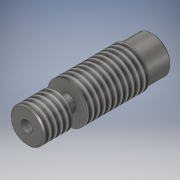
# Autodesk Inventor part: E3D-v6 1.75mm Heat Break
Saved by Autodesk Inventor 2018.2 (Build 222227000, 227)
## iProperties
Created: 2018-02-27
Part Number: E3D-v6 1.75mm Heat Break
Material: Edelstahl, 440C
Document SubType Name: Modeling
Designer: Till
Density: 7.75 g/cm^3
Appearance: Halbpoliert
Author: Till
Autodesk Inventor part; units mm, degrees
ref_plane "YZ Plane" through (0, 0, 0) normal (1, 0, 0) x (0, 1, 0)
ref_plane "XZ Plane" through (0, 0, 0) normal (0, 1, 0) x (-1, 0, 0)
ref_plane "XY Plane" through (0, 0, 0) normal (0, 0, 1) x (1, 0, 0)
sketch "Skizze1" plane through (0, 0, 0) normal (0, 0, 1) x (1, 0, 0)
  line L0 (1, 0) -> (1, 17.2649)
  line L1 (1, 17.2649) -> (2.1, 17.9)
  line L2 (2.1, 17.9) -> (2.1, 22.1)
  line L3 (2.1, 22.1) -> (3.2, 22.1)
  line L4 (3.2, 22.1) -> (3.2, 17.9)
  line L5 (3.2, 17.9) -> (3.5, 17.9)
  line L6 (3.5, 17.9) -> (3.5, 7.1)
  line L7 (3.5, 7.1) -> (1.485, 7.1)
  line L8 (1.485, 7.1) -> (1.485, 5)
  line L9 (1.485, 5) -> (3, 5)
  line L10 (3, 5) -> (3, 0)
  line L11 (3, 0) -> (1, 0)
  line L12 (0, -4.42) -> (0, 26.52) projected
  point P0 (0, 0)
  dimension "d0" = 120
  dimension "d1" = 1
  dimension "d2" = 1.485
  dimension "d3" = 0
  dimension "d4" = 5
  dimension "d5" = 2.1
  dimension "d6" = 15
  dimension "d7" = 2.1
  dimension "d8" = 3.5
  dimension "d9" = 3
  dimension "d10" = 0
  dimension "d11" = 4.2
  dimension "d12" = 3.2
  constraints: 24 end point, 9 perpendicular, 1 parallel, 1 vertical
  measures "d0" angle of L0 L1
  measures "d1" distance from line of point (0, 0) L0
  measures "d2" distance from line of point (0, 0) L8
  measures "d3" distance from line of point (0, 0) L11
  measures "d4" distance of L9.end L10.end
  measures "d5" distance of L7.end L8.end
  measures "d6" distance between parallel lines of L3 L7
  measures "d7" distance from line of point (0, 0) L2
  measures "d8" distance from line of point (0, 0) L6
  measures "d9" distance from line of point (0, 0) L10
  measures "d10" vertical distance of L5.end L1.end
  measures "d11" distance between parallel lines of L3 L5
  measures "d12" distance from line of point (0, 0) L4
revolve "Umdrehung1" add sketch "Skizze1" angle 360 about axis through (0, -10, 0) along (0, 1, 0)
chamfer "Fase1" distance 0.25 angle 45 2 edges at (-3.2, 22.1, 0) (-3, 0, 0)
thread "Gewinde1" size "M7x1" class "6g" standard "ANSI Metric M Profile" full length
thread "Gewinde2" size "M6x1" class "6g" standard "ANSI Metric M Profile" full length
